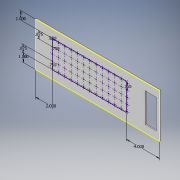
# Autodesk Inventor part: perforated side
Saved by Autodesk Inventor 2017 (Build 210142000, 142)
## iProperties
Created: 2016-10-04
Part Number: perforated side
Material: Generic
Document SubType Name: Modeling
Designer: Darien Morrow
Density: 1 g/cm^3
Appearance: Default
Author: Darien Morrow
Autodesk Inventor part; units mm, degrees
ref_plane "YZ Plane" through (0, 0, 0) normal (1, 0, 0) x (0, 1, 0)
ref_plane "XZ Plane" through (0, 0, 0) normal (0, 1, 0) x (-1, 0, 0)
ref_plane "XY Plane" through (0, 0, 0) normal (0, 0, 1) x (1, 0, 0)
sketch "Sketch1" plane through (0, 0, 0) normal (0, 0, 1) x (1, 0, 0)
  line L0 (-188.9125, -66.675) -> (188.9125, -66.675)
  line L1 (188.9125, -66.675) -> (188.9125, 66.675)
  line L2 (188.9125, 66.675) -> (-188.9125, 66.675)
  line L3 (-188.9125, 66.675) -> (-188.9125, -66.675)
  line L4 (-188.9125, -66.675) -> (188.9125, 66.675) construction
  line L5 (188.9125, -66.675) -> (-188.9125, 66.675) construction
  point P0 (0, 0)
  dimension "d0" = 133.35
  dimension "d1" = 377.825
  constraints: 12 end point, 2 midpoint, 2 parallel, 1 horizontal, 1 perpendicular
  measures "d0" distance between parallel lines of L0 L2
  measures "d1" distance between parallel lines of L1 L3
extrude "Extrusion1" add sketch "Sketch1" along normal blind 3.175
sketch "Sketch2" plane through (0, 0, 3.175) normal (0, 0, 1) x (1, 0, 0)
  line L0 (-138.1125, -41.275) -> (87.3125, -41.275)
  line L1 (87.3125, -41.275) -> (87.3125, 41.275)
  line L2 (87.3125, 41.275) -> (-138.1125, 41.275)
  line L3 (-138.1125, 41.275) -> (-138.1125, -41.275)
  line L4 (-188.9125, -66.675) -> (188.9125, -66.675) projected
  line L5 (188.9125, 66.675) -> (-188.9125, 66.675) projected
  line L6 (-188.9125, 66.675) -> (-188.9125, -66.675) projected
  line L7 (188.9125, -66.675) -> (188.9125, 66.675) projected
  point P0 (0, 0)
  point P1 (-138.1125, 19.05)
  point P2 (-138.1125, -19.05)
  point P3 (-138.1125, 0)
  point P4 (-119.0625, 19.05)
  point P5 (-119.0625, 0)
  point P6 (-119.0625, -19.05)
  point P7 (-100.0125, 19.05)
  point P8 (-100.0125, 0)
  point P9 (-100.0125, -19.05)
  point P10 (-80.9625, 19.05)
  point P11 (-80.9625, 0)
  point P12 (-80.9625, -19.05)
  point P13 (-61.9125, 19.05)
  point P14 (-61.9125, 0)
  point P15 (-61.9125, -19.05)
  point P16 (-42.8625, 19.05)
  point P17 (-42.8625, 0)
  point P18 (-42.8625, -19.05)
  point P19 (-23.8125, 19.05)
  point P20 (-23.8125, 0)
  point P21 (-23.8125, -19.05)
  point P22 (-4.7625, 19.05)
  point P23 (-4.7625, 0)
  point P24 (-4.7625, -19.05)
  point P25 (14.2875, 19.05)
  point P26 (14.2875, 0)
  point P27 (14.2875, -19.05)
  point P28 (33.3375, 19.05)
  point P29 (33.3375, 0)
  point P30 (33.3375, -19.05)
  point P31 (52.3875, 19.05)
  point P32 (52.3875, 0)
  point P33 (52.3875, -19.05)
  point P34 (71.4375, 19.05)
  point P35 (71.4375, 0)
  point P36 (71.4375, -19.05)
  point P37 (90.4875, 19.05)
  point P38 (90.4875, 0)
  point P39 (90.4875, -19.05)
  point P40 (-138.1125, -38.1)
  point P41 (-119.0625, -38.1)
  point P42 (-100.0125, -38.1)
  point P43 (-80.9625, -38.1)
  point P44 (-61.9125, -38.1)
  point P45 (-42.8625, -38.1)
  point P46 (-23.8125, -38.1)
  point P47 (-4.7625, -38.1)
  point P48 (14.2875, -38.1)
  point P49 (33.3375, -38.1)
  point P50 (52.3875, -38.1)
  point P51 (71.4375, -38.1)
  point P52 (90.4875, -38.1)
  point P53 (90.4875, 38.1)
  point P54 (71.4375, 38.1)
  point P55 (52.3875, 38.1)
  point P56 (33.3375, 38.1)
  point P57 (14.2875, 38.1)
  point P58 (-4.7625, 38.1)
  point P59 (-23.8125, 38.1)
  point P60 (-42.8625, 38.1)
  point P61 (-61.9125, 38.1)
  point P62 (-80.9625, 38.1)
  point P63 (-100.0125, 38.1)
  point P64 (-119.0625, 38.1)
  point P65 (-138.1125, 38.1)
  dimension "d4" = 25.4
  dimension "d5" = 25.4
  dimension "d6" = 50.8
  dimension "d7" = 101.6
  dimension "d8" = 22.225
  dimension "d9" = 0
  dimension "d10" = 22.225
  dimension "d13" = 19.05
  dimension "d33" = 19.05
  dimension "d40" = 19.05
  constraints: 8 end point, 2 horizontal, 2 parallel, 2 vertical, 1 midpoint, 1 perpendicular, 1 point on line, 62 other
  measures "d4" distance between parallel lines of L0 L4
  measures "d5" distance between parallel lines of L2 L5
  measures "d6" distance between parallel lines of L3 L6
  measures "d7" distance between parallel lines of L1 L7
  measures "d8" distance from line of point (-138.112, 19.05) L2
  measures "d9" distance from line of point (-138.112, 19.05) L3
  measures "d10" distance from line of point (-138.112, -19.05) L0
  measures "d13" distance of point (-138.112, 19.05) point (-119.062, 19.05)
  measures "d33" distance of point (-138.112, -19.05) point (-138.112, -38.1)
  measures "d40" distance of point (90.488, 19.05) point (90.488, 38.1)
hole "Hole1" at (-138.1125, 19.05, 3.175) at (-138.1125, -19.05, 3.175) at (-138.1125, 0, 3.175) at (-119.0625, 19.05, 3.175) at (-119.0625, 0, 3.175) at (-119.0625, -19.05, 3.175) at (-100.0125, 19.05, 3.175) at (-100.0125, 0, 3.175) at (-100.0125, -19.05, 3.175) at (-80.9625, 19.05, 3.175) at (-80.9625, 0, 3.175) at (-80.9625, -19.05, 3.175) at (-61.9125, 19.05, 3.175) at (-61.9125, 0, 3.175) at (-61.9125, -19.05, 3.175) at (-42.8625, 19.05, 3.175) at (-42.8625, 0, 3.175) at (-42.8625, -19.05, 3.175) at (-23.8125, 19.05, 3.175) at (-23.8125, 0, 3.175) at (-23.8125, -19.05, 3.175) at (-4.7625, 19.05, 3.175) at (-4.7625, 0, 3.175) at (-4.7625, -19.05, 3.175) at (14.2875, 19.05, 3.175) at (14.2875, 0, 3.175) at (14.2875, -19.05, 3.175) at (33.3375, 19.05, 3.175) at (33.3375, 0, 3.175) at (33.3375, -19.05, 3.175) at (52.3875, 19.05, 3.175) at (52.3875, 0, 3.175) at (52.3875, -19.05, 3.175) at (71.4375, 19.05, 3.175) at (71.4375, 0, 3.175) at (71.4375, -19.05, 3.175) at (90.4875, 19.05, 3.175) at (90.4875, 0, 3.175) at (90.4875, -19.05, 3.175) direction (0, 0, -1) diameter 3.175 end through all
sketch "Sketch4" plane through (0, 0, 3.175) normal (0, 0, 1) x (1, 0, 0)
  line L0 (179.3875, 44.45) -> (144.4625, 44.45)
  line L1 (144.4625, 44.45) -> (144.4625, -44.45)
  line L2 (144.4625, -44.45) -> (179.3875, -44.45)
  line L3 (179.3875, -44.45) -> (179.3875, 44.45)
  line L4 (188.9125, -66.675) -> (188.9125, 66.675) projected
  line L5 (188.9125, 66.675) -> (-188.9125, 66.675) projected
  line L6 (-188.9125, -66.675) -> (188.9125, -66.675) projected
  point P0 (0, 0)
  dimension "d25" = 9.525
  dimension "d26" = 44.45
  dimension "d27" = 22.225
  dimension "d28" = 22.225
  constraints: 8 end point, 2 parallel, 1 horizontal, 1 perpendicular
  measures "d25" distance between parallel lines of L3 L4
  measures "d26" distance between parallel lines of L4 L1
  measures "d27" distance between parallel lines of L5 L0
  measures "d28" distance between parallel lines of L2 L6
extrude "Extrusion2" cut sketch "Sketch4" against normal blind 25.4
hole "Hole2" at (-138.1125, -38.1, 3.175) at (-119.0625, -38.1, 3.175) at (-100.0125, -38.1, 3.175) at (-80.9625, -38.1, 3.175) at (-61.9125, -38.1, 3.175) at (-42.8625, -38.1, 3.175) at (-23.8125, -38.1, 3.175) at (-4.7625, -38.1, 3.175) at (14.2875, -38.1, 3.175) at (33.3375, -38.1, 3.175) at (52.3875, -38.1, 3.175) at (71.4375, -38.1, 3.175) at (90.4875, -38.1, 3.175) at (90.4875, 38.1, 3.175) at (71.4375, 38.1, 3.175) at (52.3875, 38.1, 3.175) at (33.3375, 38.1, 3.175) at (14.2875, 38.1, 3.175) at (-4.7625, 38.1, 3.175) at (-23.8125, 38.1, 3.175) at (-42.8625, 38.1, 3.175) at (-61.9125, 38.1, 3.175) at (-80.9625, 38.1, 3.175) at (-100.0125, 38.1, 3.175) at (-119.0625, 38.1, 3.175) at (-138.1125, 38.1, 3.175) direction (0, 0, -1) diameter 3.175 end through all
body "Solid1"
